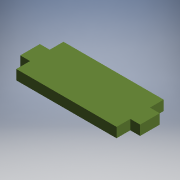
# Autodesk Inventor part: Middle_leg_c
Saved by Autodesk Inventor 2017 (Build 210142000, 142)
## iProperties
Part Number: Middle_leg_c
Material: Generic
Document SubType Name: Modeling
Designer: Alexander Miller
Appearance: Olive Green
Author: Alexander Miller
Autodesk Inventor part; units mm, degrees
ref_plane "YZ Plane" through (0, 0, 0) normal (1, 0, 0) x (0, 1, 0)
ref_plane "XZ Plane" through (0, 0, 0) normal (0, 1, 0) x (-1, 0, 0)
ref_plane "XY Plane" through (0, 0, 0) normal (0, 0, 1) x (1, 0, 0)
sketch "Sketch1" plane through (0, 0, 0) normal (0, 1, 0) x (-1, 0, 0)
  line L0 (25.5, 12) -> (-25.5, 12)
  line L1 (-25.5, 12) -> (-25.5, -12)
  line L2 (-25.5, -12) -> (25.5, -12)
  line L3 (25.5, -12) -> (25.5, 12)
  line L4 (42.7, 0) -> (-42.7, 0) projected
  line L5 (0, -16.8) -> (0, 16.8) projected
  line L6 (25.5, -5) -> (30.5, -5)
  line L7 (30.5, -5) -> (30.5, 5)
  line L8 (30.5, 5) -> (25.5, 5)
  line L9 (25.5, 5) -> (25.5, -5)
  line L10 (-25.5, -5) -> (-30.5, -5)
  line L11 (-30.5, -5) -> (-30.5, 5)
  line L12 (-30.5, 5) -> (-25.5, 5)
  line L13 (-25.5, 5) -> (-25.5, -5)
  point P0 (0, 0)
  point P1 (0, 12)
  point P2 (30.5, 0)
  point P3 (25.5, 0)
  point P4 (-25.5, 7)
  point P5 (-30.5, 0)
  point P6 (-25.5, 0)
  dimension "d3" = 24
  dimension "d4" = 51
  dimension "d7" = 5
  dimension "d8" = 10
  constraints: 24 end point, 6 symmetric about line, 4 parallel, 3 midpoint, 2 horizontal, 2 horizontal alignment, 2 perpendicular, 1 point on line, 1 vertical alignment
  measures "d3" distance of L2.end L0.start
  measures "d4" distance between parallel lines of L1 L3
  measures "d7" distance of L6.start L6.end
  measures "d8" distance of L6.end L7.end
extrude "Extrusion1" add sketch "Sketch1" along normal blind 5
equation "\"d3\" = sa_diameter"
equation "\"d4\" = b_mat_thickness + s_shaft_height + s_height + sa_thickness"
equation "\"d7\" = b_mat_thickness"
equation "\"d5\" = b_mat_thickness"
equation "\"sa_diameter\" = 24"
equation "\"b_mat_thickness\" = 5"
equation "\"s_shaft_height\" = 6"
equation "\"s_height\" = 38"
equation "\"sa_thickness\" = 2"
body "Solid1"
